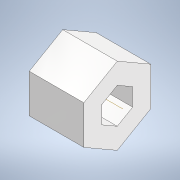
# Autodesk Inventor part: Adaptador Acoplador
Saved by Autodesk Inventor 2020.3 (Build 243373000, 373)
## iProperties
Created: 2020-11-02
Part Number: Adaptador Acoplador
Material: ABS Plastic
Document SubType Name: Modeling
Designer: juanp
Density: 1.06 g/cm^3
Appearance: Smooth - White
Mass: 0.556594 g
Surface Area: 5.27565 cm^2
Volume: 0.525089 cm^3
Author: juanp
Autodesk Inventor part; units mm, degrees
ref_plane "YZ Plane" through (0, 0, 0) normal (1, 0, 0) x (0, 1, 0)
ref_plane "XZ Plane" through (0, 0, 0) normal (0, 1, 0) x (-1, 0, 0)
ref_plane "XY Plane" through (0, 0, 0) normal (0, 0, 1) x (1, 0, 0)
sketch "Sketch1" plane through (0, 0, 0) normal (1, 0, 0) x (0, 1, 0)
  line L0 (-1.299, -2.25) -> (-2.5981, 0)
  line L1 (-2.5981, 0) -> (-1.299, 2.25)
  line L2 (-1.299, 2.25) -> (1.299, 2.25)
  line L3 (1.299, 2.25) -> (2.5981, 0)
  line L4 (2.5981, 0) -> (1.299, -2.25)
  line L5 (1.299, -2.25) -> (-1.299, -2.25)
  line L6 (-2.829, -4.9) -> (-5.658, 0)
  line L7 (-5.658, 0) -> (-2.829, 4.9)
  line L8 (-2.829, 4.9) -> (2.829, 4.9)
  line L9 (2.829, 4.9) -> (5.658, 0)
  line L10 (5.658, 0) -> (2.829, -4.9)
  line L11 (2.829, -4.9) -> (-2.829, -4.9)
  point P0 (0, 0)
  point P1 (0, 0)
  point P2 (0, 0)
  dimension "d0" = 4.5
  dimension "d1" = 9.8
  constraints: 24 end point, 2 coincident, 1 horizontal, 1 parallel, 26 other
  measures "d0" distance between parallel lines of L2 L5
  measures "d1" distance between parallel lines of L11 L8
extrude "Extrusion1" add sketch "Sketch1" along normal blind 8
body "Solid1"
